Autodesk Inventor part; units mm, degrees
(part 4 of 8)
  arc A302 (101.3786, 36.5166) -> (101.4167, 36.5166) centre (101.3976, 36.5166) ccw
  arc A303 (101.1627, 36.7706) -> (101.1627, 36.7325) centre (101.1627, 36.7516) ccw
  arc A304 (101.1627, 36.7515) -> (100.8756, 36.5427) centre (101.1627, 36.4497) ccw
  arc A305 (101.1627, 36.7325) -> (101.1627, 36.7706) centre (101.1627, 36.7516) ccw
  arc A306 (100.8574, 36.5486) -> (100.8937, 36.5368) centre (100.8756, 36.5427) ccw
  arc A307 (101.3194, 36.3338) -> (101.3977, 36.5166) centre (101.1452, 36.5166) ccw
  arc A308 (101.3062, 36.3476) -> (101.3325, 36.32) centre (101.3194, 36.3338) ccw
  arc A309 (101.4167, 36.5166) -> (101.3786, 36.5166) centre (101.3976, 36.5166) ccw
  line L109 (101.3194, 36.3338) -> (100.8756, 35.8117)
  arc A310 (100.8611, 35.8241) -> (100.8901, 35.7994) centre (100.8756, 35.8118) ccw
  arc A311 (101.3339, 36.3215) -> (101.3049, 36.3462) centre (101.3194, 36.3338) ccw
  line L110 (100.8756, 35.8117) -> (101.3977, 35.8117)
  arc A312 (101.3977, 35.7927) -> (101.3977, 35.8308) centre (101.3977, 35.8118) ccw
  arc A313 (100.8756, 35.8308) -> (100.8756, 35.7927) centre (100.8756, 35.8118) ccw
  arc A314 (98.4358, 24.7896) -> (98.4358, 40.7896) centre (98.4358, 32.7896) ccw
  arc A315 (98.4358, 40.7896) -> (98.4358, 24.7896) centre (98.4358, 32.7896) ccw
  arc A316 (98.4358, 26.2704) -> (98.4358, 39.3088) centre (98.4358, 32.7896) ccw
  arc A317 (98.4358, 39.3088) -> (98.4358, 26.2704) centre (98.4358, 32.7896) ccw
  arc A318 (98.4358, 23.2896) -> (98.4358, 42.2896) centre (98.4358, 32.7896) ccw
  arc A319 (98.4358, 42.2896) -> (98.4358, 23.2896) centre (98.4358, 32.7896) ccw
  arc A320 (75.8576, 81.3321) -> (77.8576, 81.3321) centre (76.8576, 81.3321) ccw
  arc A321 (75.8893, 81.3321) -> (75.8258, 81.3321) centre (75.8576, 81.3321) ccw
  arc A322 (77.8893, 81.3321) -> (77.8258, 81.3321) centre (77.8576, 81.3321) ccw
  line L111 (73.2973, 78.5852) -> (73.5584, 78.794)
  arc A323 (73.5703, 78.7791) -> (73.5465, 78.8089) centre (73.5584, 78.794) ccw
  arc A324 (73.2854, 78.6) -> (73.3092, 78.5703) centre (73.2973, 78.5851) ccw
  line L112 (73.5584, 78.794) -> (73.5584, 77.8542)
  arc A325 (73.5394, 77.8542) -> (73.5774, 77.8542) centre (73.5584, 77.8542) ccw
  arc A326 (73.5774, 78.794) -> (73.5394, 78.794) centre (73.5584, 78.794) ccw
  line L113 (73.2973, 77.8542) -> (73.8195, 77.8542)
  arc A327 (73.8195, 77.8352) -> (73.8195, 77.8732) centre (73.8195, 77.8542) ccw
  arc A328 (73.2973, 77.8732) -> (73.2973, 77.8352) centre (73.2973, 77.8542) ccw
  arc A329 (79.8195, 78.559) -> (79.5845, 78.794) centre (79.5845, 78.559) ccw
  arc A330 (79.8004, 78.559) -> (79.8385, 78.559) centre (79.8194, 78.559) ccw
  arc A331 (79.5845, 78.813) -> (79.5845, 78.775) centre (79.5845, 78.794) ccw
  arc A332 (79.5845, 78.794) -> (79.2973, 78.5852) centre (79.5844, 78.4922) ccw
  arc A333 (79.5845, 78.775) -> (79.5845, 78.813) centre (79.5845, 78.794) ccw
  arc A334 (79.2792, 78.591) -> (79.3155, 78.5793) centre (79.2973, 78.5851) ccw
  arc A335 (79.7411, 78.3763) -> (79.8195, 78.559) centre (79.5671, 78.5591) ccw
  arc A336 (79.728, 78.3901) -> (79.7543, 78.3625) centre (79.7412, 78.3763) ccw
  arc A337 (79.8385, 78.559) -> (79.8004, 78.5591) centre (79.8194, 78.559) ccw
  line L114 (79.7411, 78.3763) -> (79.2973, 77.8542)
  arc A338 (79.2828, 77.8665) -> (79.3119, 77.8419) centre (79.2973, 77.8542) ccw
  arc A339 (79.7557, 78.364) -> (79.7266, 78.3886) centre (79.7412, 78.3763) ccw
  line L115 (79.2973, 77.8542) -> (79.8195, 77.8542)
  arc A340 (79.8195, 77.8352) -> (79.8195, 77.8732) centre (79.8195, 77.8542) ccw
  arc A341 (79.2973, 77.8732) -> (79.2973, 77.8352) centre (79.2973, 77.8542) ccw
  arc A342 (76.8576, 66.8321) -> (76.8576, 82.8321) centre (76.8576, 74.8321) ccw
  arc A343 (76.8576, 82.8321) -> (76.8576, 66.8321) centre (76.8576, 74.8321) ccw
  arc A344 (76.8576, 68.3129) -> (76.8576, 81.3513) centre (76.8576, 74.8321) ccw
  arc A345 (76.8576, 81.3513) -> (76.8576, 68.3129) centre (76.8576, 74.8321) ccw
  arc A346 (76.8576, 65.3321) -> (76.8576, 84.3321) centre (76.8576, 74.8321) ccw
  arc A347 (97.4424, 81.3321) -> (99.4424, 81.3321) centre (98.4424, 81.3321) ccw
  arc A348 (97.4741, 81.3321) -> (97.4106, 81.3321) centre (97.4424, 81.3321) ccw
  arc A349 (99.4741, 81.3321) -> (99.4106, 81.3321) centre (99.4424, 81.3321) ccw
  line L116 (94.8822, 78.5852) -> (95.1432, 78.794)
  arc A350 (95.1551, 78.7791) -> (95.1313, 78.8089) centre (95.1432, 78.794) ccw
  arc A351 (94.8703, 78.6) -> (94.8941, 78.5703) centre (94.8822, 78.5851) ccw
  line L117 (95.1432, 78.794) -> (95.1432, 77.8542)
  arc A352 (95.1242, 77.8542) -> (95.1623, 77.8542) centre (95.1432, 77.8542) ccw
  arc A353 (95.1623, 78.794) -> (95.1242, 78.794) centre (95.1432, 78.794) ccw
  line L118 (94.8822, 77.8542) -> (95.4043, 77.8542)
  arc A354 (95.4043, 77.8352) -> (95.4043, 77.8732) centre (95.4043, 77.8542) ccw
  arc A355 (94.8822, 77.8732) -> (94.8822, 77.8352) centre (94.8822, 77.8542) ccw
  arc A356 (101.4043, 78.559) -> (101.1693, 78.794) centre (101.1693, 78.559) ccw
  arc A357 (101.3852, 78.559) -> (101.4233, 78.559) centre (101.4043, 78.559) ccw
  arc A358 (101.1693, 78.813) -> (101.1693, 78.775) centre (101.1693, 78.794) ccw
  arc A359 (101.1693, 78.794) -> (100.8822, 78.5852) centre (101.1693, 78.4922) ccw
  arc A360 (101.1693, 78.775) -> (101.1693, 78.813) centre (101.1693, 78.794) ccw
  arc A361 (100.864, 78.591) -> (100.9003, 78.5793) centre (100.8821, 78.5851) ccw
  arc A362 (101.326, 78.3763) -> (101.4043, 78.559) centre (101.1519, 78.559) ccw
  arc A363 (101.3128, 78.3901) -> (101.3391, 78.3625) centre (101.326, 78.3763) ccw
  arc A364 (101.4233, 78.559) -> (101.3852, 78.5591) centre (101.4043, 78.559) ccw
  line L119 (101.326, 78.3763) -> (100.8822, 77.8542)
  arc A365 (100.8677, 77.8665) -> (100.8967, 77.8419) centre (100.8822, 77.8542) ccw
  arc A366 (101.3405, 78.364) -> (101.3114, 78.3886) centre (101.326, 78.3763) ccw
  line L120 (100.8822, 77.8542) -> (101.4043, 77.8542)
  arc A367 (101.4043, 77.8352) -> (101.4043, 77.8732) centre (101.4043, 77.8542) ccw
  arc A368 (100.8822, 77.8732) -> (100.8822, 77.8352) centre (100.8822, 77.8542) ccw
  arc A369 (98.4424, 66.8321) -> (98.4424, 82.8321) centre (98.4424, 74.8321) ccw
  arc A370 (98.4424, 82.8321) -> (98.4424, 66.8321) centre (98.4424, 74.8321) ccw
  arc A371 (98.4424, 68.3129) -> (98.4424, 81.3513) centre (98.4424, 74.8321) ccw
  arc A372 (98.4424, 81.3513) -> (98.4424, 68.3129) centre (98.4424, 74.8321) ccw
  arc A373 (98.4424, 65.3321) -> (98.4424, 84.3321) centre (98.4424, 74.8321) ccw
  arc A374 (98.4424, 84.3321) -> (98.4424, 65.3321) centre (98.4424, 74.8321) ccw
  arc A375 (34.6796, 5.5886) -> (32.6796, 5.5886) centre (33.6796, 5.5886) ccw
  arc A376 (34.6479, 5.5886) -> (34.7114, 5.5886) centre (34.6796, 5.5886) ccw
  arc A377 (32.6479, 5.5886) -> (32.7114, 5.5886) centre (32.6796, 5.5886) ccw
  line L121 (38.7177, 11.8577) -> (38.9788, 12.0665)
  arc A378 (38.9907, 12.0517) -> (38.9669, 12.0814) centre (38.9788, 12.0665) ccw
  arc A379 (38.7058, 11.8726) -> (38.7296, 11.8428) centre (38.7177, 11.8577) ccw
  line L122 (38.9788, 12.0665) -> (38.9788, 11.1267)
  arc A380 (38.9597, 11.1267) -> (38.9978, 11.1267) centre (38.9787, 11.1267) ccw
  arc A381 (38.9978, 12.0665) -> (38.9597, 12.0665) centre (38.9787, 12.0665) ccw
  line L123 (38.7177, 11.1267) -> (39.2398, 11.1267)
  arc A382 (39.2398, 11.1077) -> (39.2398, 11.1458) centre (39.2398, 11.1268) ccw
  arc A383 (38.7177, 11.1458) -> (38.7177, 11.1077) centre (38.7177, 11.1268) ccw
  arc A384 (36.2398, 16.8316) -> (36.0049, 17.0665) centre (36.0049, 16.8316) ccw
  arc A385 (36.2208, 16.8316) -> (36.2589, 16.8316) centre (36.2398, 16.8316) ccw
  arc A386 (36.0049, 17.0856) -> (36.0049, 17.0475) centre (36.0049, 17.0665) ccw
  arc A387 (36.0049, 17.0665) -> (35.7177, 16.8577) centre (36.0048, 16.7647) ccw
  arc A388 (36.0049, 17.0475) -> (36.0049, 17.0856) centre (36.0049, 17.0665) ccw
  arc A389 (35.6996, 16.8636) -> (35.7358, 16.8518) centre (35.7177, 16.8577) ccw
  arc A390 (36.1615, 16.6488) -> (36.2398, 16.8316) centre (35.9873, 16.8316) ccw
  arc A391 (36.1484, 16.6626) -> (36.1746, 16.635) centre (36.1615, 16.6488) ccw
  arc A392 (36.2589, 16.8316) -> (36.2208, 16.8316) centre (36.2398, 16.8316) ccw
  line L124 (36.1615, 16.6488) -> (35.7177, 16.1267)
  arc A393 (35.7032, 16.1391) -> (35.7322, 16.1144) centre (35.7177, 16.1268) ccw
  arc A394 (36.176, 16.6365) -> (36.147, 16.6612) centre (36.1615, 16.6489) ccw
  line L125 (35.7177, 16.1267) -> (36.2398, 16.1267)
  arc A395 (36.2398, 16.1077) -> (36.2398, 16.1458) centre (36.2398, 16.1268) ccw
  arc A396 (35.7177, 16.1458) -> (35.7177, 16.1077) centre (35.7177, 16.1268) ccw
  line L126 (32.7177, 11.1267) -> (32.9788, 11.1267)
  arc A397 (32.9788, 11.1077) -> (32.9788, 11.1458) centre (32.9788, 11.1268) ccw
  arc A398 (32.7177, 11.1458) -> (32.7177, 11.1077) centre (32.7177, 11.1268) ccw
  arc A399 (32.9788, 11.1267) -> (32.9788, 11.6488) centre (32.9788, 11.3878) ccw
  arc A400 (32.9788, 11.1458) -> (32.9788, 11.1077) centre (32.9788, 11.1268) ccw
  arc A401 (32.9788, 11.6679) -> (32.9788, 11.6298) centre (32.9788, 11.6488) ccw
  line L127 (32.7177, 12.0665) -> (33.031, 12.0665)
  arc A402 (33.031, 12.0475) -> (33.031, 12.0856) centre (33.031, 12.0665) ccw
  arc A403 (32.7177, 12.0856) -> (32.7177, 12.0475) centre (32.7177, 12.0665) ccw
  arc A404 (33.031, 11.6488) -> (33.031, 12.0665) centre (33.031, 11.8576) ccw
  arc A405 (33.031, 11.6679) -> (33.031, 11.6298) centre (33.031, 11.6488) ccw
  arc A406 (33.031, 12.0856) -> (33.031, 12.0475) centre (33.031, 12.0665) ccw
  line L128 (33.031, 11.6488) -> (32.8221, 11.6488)
  arc A407 (32.8221, 11.6679) -> (32.8221, 11.6298) centre (32.8221, 11.6488) ccw
  arc A408 (33.031, 11.6298) -> (33.031, 11.6679) centre (33.031, 11.6488) ccw
  arc A409 (33.6796, 4.0886) -> (33.6796, 20.0886) centre (33.6796, 12.0886) ccw
  arc A410 (33.6796, 20.0886) -> (33.6796, 4.0886) centre (33.6796, 12.0886) ccw
  arc A411 (33.6796, 5.5694) -> (33.6796, 18.6078) centre (33.6796, 12.0886) ccw
  arc A412 (33.6796, 18.6078) -> (33.6796, 5.5694) centre (33.6796, 12.0886) ccw
  arc A413 (33.6796, 2.5886) -> (33.6796, 21.5886) centre (33.6796, 12.0886) ccw
  arc A414 (33.6796, 21.5886) -> (33.6796, 2.5886) centre (33.6796, 12.0886) ccw
  arc A415 (32.6842, 60.4569) -> (34.6842, 60.4569) centre (33.6842, 60.4569) ccw
  arc A416 (32.716, 60.4569) -> (32.6525, 60.4569) centre (32.6843, 60.4569) ccw
  arc A417 (34.716, 60.4569) -> (34.6525, 60.4569) centre (34.6843, 60.4569) ccw
  line L129 (28.624, 55.21) -> (28.8851, 55.4188)
  arc A418 (28.897, 55.4039) -> (28.8732, 55.4337) centre (28.8851, 55.4188) ccw
  arc A419 (28.6121, 55.2248) -> (28.6359, 55.1951) centre (28.624, 55.2099) ccw
  line L130 (28.8851, 55.4188) -> (28.8851, 54.479)
  arc A420 (28.866, 54.479) -> (28.9041, 54.479) centre (28.8851, 54.479) ccw
  arc A421 (28.9041, 55.4188) -> (28.866, 55.4188) centre (28.8851, 55.4188) ccw
  line L131 (28.624, 54.479) -> (29.1461, 54.479)
  arc A422 (29.1461, 54.46) -> (29.1461, 54.4981) centre (29.1461, 54.4791) ccw
  arc A423 (28.624, 54.4981) -> (28.624, 54.46) centre (28.624, 54.4791) ccw
  arc A424 (29.1461, 53.1839) -> (28.9112, 53.4188) centre (28.9112, 53.1839) ccw
  arc A425 (29.1271, 53.1839) -> (29.1652, 53.1839) centre (29.1461, 53.1839) ccw
  arc A426 (28.9112, 53.4379) -> (28.9112, 53.3998) centre (28.9112, 53.4189) ccw
  arc A427 (28.9112, 53.4188) -> (28.624, 53.21) centre (28.9111, 53.117) ccw
  arc A428 (28.9112, 53.3998) -> (28.9112, 53.4379) centre (28.9112, 53.4189) ccw
  arc A429 (28.6059, 53.2158) -> (28.6421, 53.2041) centre (28.624, 53.2099) ccw
  arc A430 (29.0678, 53.0011) -> (29.1461, 53.1839) centre (28.8936, 53.1839) ccw
  arc A431 (29.0547, 53.0149) -> (29.0809, 52.9873) centre (29.0678, 53.0011) ccw
  arc A432 (29.1652, 53.1839) -> (29.1271, 53.1839) centre (29.1461, 53.1839) ccw
  line L132 (29.0678, 53.0011) -> (28.624, 52.479)
  arc A433 (28.6095, 52.4914) -> (28.6385, 52.4667) centre (28.624, 52.4791) ccw
  arc A434 (29.0823, 52.9888) -> (29.0533, 53.0135) centre (29.0678, 53.0011) ccw
  line L133 (28.624, 52.479) -> (29.1461, 52.479)
  arc A435 (29.1461, 52.46) -> (29.1461, 52.4981) centre (29.1461, 52.4791) ccw
  arc A436 (28.624, 52.4981) -> (28.624, 52.46) centre (28.624, 52.4791) ccw
  line L134 (38.124, 52.479) -> (38.3851, 52.479)
  arc A437 (38.3851, 52.46) -> (38.3851, 52.4981) centre (38.3851, 52.4791) ccw
  arc A438 (38.124, 52.4981) -> (38.124, 52.46) centre (38.124, 52.4791) ccw
  arc A439 (38.3851, 52.479) -> (38.3851, 53.0011) centre (38.3851, 52.74) ccw
  arc A440 (38.3851, 52.4981) -> (38.3851, 52.46) centre (38.3851, 52.4791) ccw
  arc A441 (38.3851, 53.0202) -> (38.3851, 52.9821) centre (38.3851, 53.0012) ccw
  line L135 (38.124, 53.4188) -> (38.4373, 53.4188)
  arc A442 (38.4373, 53.3998) -> (38.4373, 53.4379) centre (38.4373, 53.4189) ccw
  arc A443 (38.124, 53.4379) -> (38.124, 53.3998) centre (38.124, 53.4189) ccw
  arc A444 (38.4373, 53.0011) -> (38.4373, 53.4188) centre (38.4373, 53.2099) ccw
  arc A445 (38.4373, 53.0202) -> (38.4373, 52.9821) centre (38.4373, 53.0012) ccw
  arc A446 (38.4373, 53.4379) -> (38.4373, 53.3998) centre (38.4373, 53.4189) ccw
  line L136 (38.4373, 53.0011) -> (38.2284, 53.0011)
  arc A447 (38.2284, 53.0202) -> (38.2284, 52.9821) centre (38.2284, 53.0012) ccw
  arc A448 (38.4373, 52.9821) -> (38.4373, 53.0202) centre (38.4373, 53.0012) ccw
  line L137 (38.3328, 55.4188) -> (38.124, 54.6879)
  arc A449 (38.1057, 54.6931) -> (38.1423, 54.6826) centre (38.124, 54.6879) ccw
  arc A450 (38.3512, 55.4136) -> (38.3145, 55.424) centre (38.3329, 55.4188) ccw
  line L138 (38.124, 54.6879) -> (38.6461, 54.6879)
  arc A451 (38.6461, 54.6688) -> (38.6461, 54.7069) centre (38.6461, 54.6879) ccw
  arc A452 (38.124, 54.7069) -> (38.124, 54.6688) centre (38.124, 54.6879) ccw
  line L139 (38.4895, 54.8967) -> (38.4895, 54.479)
  arc A453 (38.4704, 54.479) -> (38.5085, 54.479) centre (38.4894, 54.479) ccw
  arc A454 (38.5085, 54.8967) -> (38.4704, 54.8967) centre (38.4894, 54.8967) ccw
  arc A455 (33.6842, 45.9569) -> (33.6842, 61.9569) centre (33.6842, 53.9569) ccw
  arc A456 (33.6842, 61.9569) -> (33.6842, 45.9569) centre (33.6842, 53.9569) ccw
  arc A457 (33.6842, 47.4377) -> (33.6842, 60.4761) centre (33.6842, 53.9569) ccw
  arc A458 (33.6842, 60.4761) -> (33.6842, 47.4377) centre (33.6842, 53.9569) ccw
  arc A459 (33.6842, 44.4569) -> (33.6842, 63.4569) centre (33.6842, 53.9569) ccw
  arc A460 (33.6842, 63.4569) -> (33.6842, 44.4569) centre (33.6842, 53.9569) ccw
  arc A461 (11.0477, 60.2972) -> (13.0477, 60.2972) centre (12.0477, 60.2972) ccw
  arc A462 (11.0794, 60.2972) -> (11.0159, 60.2972) centre (11.0477, 60.2972) ccw
  arc A463 (13.0794, 60.2972) -> (13.0159, 60.2972) centre (13.0477, 60.2972) ccw
  line L140 (6.4875, 54.5503) -> (6.7485, 54.7591)
  arc A464 (6.7604, 54.7442) -> (6.7366, 54.774) centre (6.7485, 54.7591) ccw
  arc A465 (6.4756, 54.5651) -> (6.4994, 54.5354) centre (6.4875, 54.5503) ccw
  line L141 (6.7485, 54.7591) -> (6.7485, 53.8193)
  arc A466 (6.7295, 53.8193) -> (6.7676, 53.8193) centre (6.7485, 53.8193) ccw
  arc A467 (6.7676, 54.7591) -> (6.7295, 54.7591) centre (6.7485, 54.7591) ccw
  line L142 (6.4875, 53.8193) -> (7.0096, 53.8193)
  arc A468 (7.0096, 53.8003) -> (7.0096, 53.8384) centre (7.0096, 53.8194) ccw
  arc A469 (6.4875, 53.8384) -> (6.4875, 53.8003) centre (6.4875, 53.8194) ccw
  arc A470 (10.0096, 49.5242) -> (9.7746, 49.7591) centre (9.7746, 49.5241) ccw
  arc A471 (9.9905, 49.5242) -> (10.0286, 49.5242) centre (10.0096, 49.5242) ccw
  arc A472 (9.7746, 49.7782) -> (9.7746, 49.7401) centre (9.7746, 49.7592) ccw
  arc A473 (9.7746, 49.7591) -> (9.4875, 49.5503) centre (9.7746, 49.4573) ccw
  arc A474 (9.7746, 49.7401) -> (9.7746, 49.7781) centre (9.7746, 49.7591) ccw
  arc A475 (9.4694, 49.5561) -> (9.5056, 49.5444) centre (9.4875, 49.5503) ccw
  arc A476 (9.9313, 49.3414) -> (10.0096, 49.5242) centre (9.7571, 49.5242) ccw
  arc A477 (9.9181, 49.3552) -> (9.9444, 49.3276) centre (9.9313, 49.3414) ccw
  arc A478 (10.0286, 49.5241) -> (9.9905, 49.5242) centre (10.0096, 49.5242) ccw
  line L143 (9.9313, 49.3414) -> (9.4875, 48.8193)
  arc A479 (9.473, 48.8316) -> (9.502, 48.807) centre (9.4875, 48.8193) ccw
  arc A480 (9.9458, 49.3291) -> (9.9168, 49.3537) centre (9.9313, 49.3414) ccw
  line L144 (9.4875, 48.8193) -> (10.0096, 48.8193)
  arc A481 (10.0096, 48.8003) -> (10.0096, 48.8384) centre (10.0096, 48.8194) ccw
  arc A482 (9.4875, 48.8384) -> (9.4875, 48.8003) centre (9.4875, 48.8194) ccw
  line L145 (12.4875, 53.8193) -> (12.7485, 53.8193)
  arc A483 (12.7485, 53.8003) -> (12.7485, 53.8384) centre (12.7485, 53.8194) ccw
  arc A484 (12.4875, 53.8384) -> (12.4875, 53.8003) centre (12.4875, 53.8194) ccw
  arc A485 (12.7485, 53.8193) -> (12.7485, 54.3414) centre (12.7485, 54.0803) ccw
  arc A486 (12.7485, 53.8384) -> (12.7485, 53.8003) centre (12.7485, 53.8194) ccw
  arc A487 (12.7485, 54.3605) -> (12.7485, 54.3224) centre (12.7485, 54.3415) ccw
  line L146 (12.4875, 54.7591) -> (12.8007, 54.7591)
  arc A488 (12.8007, 54.7401) -> (12.8007, 54.7782) centre (12.8007, 54.7592) ccw
  arc A489 (12.4875, 54.7782) -> (12.4875, 54.7401) centre (12.4875, 54.7592) ccw
  arc A490 (12.8007, 54.3414) -> (12.8007, 54.7591) centre (12.8007, 54.5502) ccw
  arc A491 (12.8007, 54.3605) -> (12.8007, 54.3224) centre (12.8007, 54.3415) ccw
  arc A492 (12.8007, 54.7782) -> (12.8007, 54.7401) centre (12.8007, 54.7592) ccw
  line L147 (12.8007, 54.3414) -> (12.5919, 54.3414)
  arc A493 (12.5919, 54.3605) -> (12.5919, 54.3224) centre (12.5919, 54.3415) ccw
  arc A494 (12.8007, 54.3224) -> (12.8007, 54.3605) centre (12.8007, 54.3415) ccw
  arc A495 (12.0477, 45.7972) -> (12.0477, 61.7972) centre (12.0477, 53.7972) ccw
  arc A496 (12.0477, 61.7972) -> (12.0477, 45.7972) centre (12.0477, 53.7972) ccw
  arc A497 (12.0477, 47.278) -> (12.0477, 60.3164) centre (12.0477, 53.7972) ccw
  arc A498 (12.0477, 60.3164) -> (12.0477, 47.278) centre (12.0477, 53.7972) ccw
  arc A499 (12.0477, 44.2972) -> (12.0477, 63.2972) centre (12.0477, 53.7972) ccw
  arc A500 (12.0477, 63.2972) -> (12.0477, 44.2972) centre (12.0477, 53.7972) ccw
  arc A501 (13.085, 5.5469) -> (11.085, 5.5469) centre (12.085, 5.5469) ccw
  arc A502 (13.0532, 5.5469) -> (13.1167, 5.5469) centre (13.0849, 5.5469) ccw
  arc A503 (11.0532, 5.5469) -> (11.1167, 5.5469) centre (11.0849, 5.5469) ccw
  line L148 (17.1231, 11.816) -> (17.3842, 12.0248)
  arc A504 (17.3961, 12.0099) -> (17.3722, 12.0397) centre (17.3841, 12.0248) ccw
  arc A505 (17.1112, 11.8308) -> (17.135, 11.8011) centre (17.1231, 11.816) ccw
  line L149 (17.3842, 12.0248) -> (17.3842, 11.085)
  arc A506 (17.3651, 11.085) -> (17.4032, 11.085) centre (17.3841, 11.085) ccw
  arc A507 (17.4032, 12.0248) -> (17.3651, 12.0248) centre (17.3841, 12.0248) ccw
  line L150 (17.1231, 11.085) -> (17.6452, 11.085)
  arc A508 (17.6452, 11.066) -> (17.6452, 11.1041) centre (17.6452, 11.0851) ccw
  arc A509 (17.1231, 11.1041) -> (17.1231, 11.066) centre (17.1231, 11.0851) ccw
  arc A510 (14.6452, 16.7899) -> (14.4103, 17.0248) centre (14.4103, 16.7899) ccw
  arc A511 (14.6262, 16.7899) -> (14.6643, 16.7899) centre (14.6453, 16.7899) ccw
  arc A512 (14.4103, 17.0439) -> (14.4103, 17.0058) centre (14.4103, 17.0249) ccw
  arc A513 (14.4103, 17.0248) -> (14.1231, 16.816) centre (14.4102, 16.723) ccw
  arc A514 (14.4103, 17.0058) -> (14.4103, 17.0439) centre (14.4103, 17.0249) ccw
  arc A515 (14.105, 16.8218) -> (14.1412, 16.8101) centre (14.1231, 16.816) ccw
  arc A516 (14.5669, 16.6071) -> (14.6452, 16.7899) centre (14.3927, 16.7899) ccw
  arc A517 (14.5538, 16.6209) -> (14.58, 16.5933) centre (14.5669, 16.6071) ccw
  arc A518 (14.6643, 16.7899) -> (14.6262, 16.7899) centre (14.6453, 16.7899) ccw
  line L151 (14.5669, 16.6071) -> (14.1231, 16.085)
  arc A519 (14.1086, 16.0974) -> (14.1376, 16.0727) centre (14.1231, 16.0851) ccw
  arc A520 (14.5814, 16.5948) -> (14.5524, 16.6195) centre (14.5669, 16.6071) ccw
  line L152 (14.1231, 16.085) -> (14.6452, 16.085)
  arc A521 (14.6452, 16.066) -> (14.6452, 16.1041) centre (14.6452, 16.0851) ccw
  arc A522 (14.1231, 16.1041) -> (14.1231, 16.066) centre (14.1231, 16.0851) ccw
  line L153 (11.1231, 11.085) -> (11.3841, 11.085)
  arc A523 (11.3841, 11.066) -> (11.3841, 11.1041) centre (11.3841, 11.0851) ccw
  arc A524 (11.1231, 11.1041) -> (11.1231, 11.066) centre (11.1231, 11.0851) ccw
  arc A525 (11.3841, 11.085) -> (11.3841, 11.6071) centre (11.3841, 11.3461) ccw
  arc A526 (11.3841, 11.1041) -> (11.3841, 11.066) centre (11.3841, 11.0851) ccw
  arc A527 (11.3841, 11.6262) -> (11.3841, 11.5881) centre (11.3841, 11.6072) ccw
  line L154 (11.1231, 12.0248) -> (11.4364, 12.0248)
  arc A528 (11.4364, 12.0058) -> (11.4364, 12.0439) centre (11.4364, 12.0249) ccw
  arc A529 (11.1231, 12.0439) -> (11.1231, 12.0058) centre (11.1231, 12.0249) ccw
  arc A530 (11.4364, 11.6071) -> (11.4364, 12.0248) centre (11.4364, 11.816) ccw
  arc A531 (11.4364, 11.6262) -> (11.4364, 11.5881) centre (11.4364, 11.6072) ccw
  arc A532 (11.4364, 12.0439) -> (11.4364, 12.0058) centre (11.4364, 12.0249) ccw
  line L155 (11.4364, 11.6071) -> (11.2275, 11.6071)
  arc A533 (11.2275, 11.6262) -> (11.2275, 11.5881) centre (11.2275, 11.6072) ccw
  arc A534 (11.4364, 11.5881) -> (11.4364, 11.6262) centre (11.4364, 11.6072) ccw
  arc A535 (12.085, 4.0469) -> (12.085, 20.0469) centre (12.085, 12.0469) ccw
  arc A536 (12.085, 20.0469) -> (12.085, 4.0469) centre (12.085, 12.0469) ccw
  arc A537 (12.085, 5.5277) -> (12.085, 18.5661) centre (12.085, 12.0469) ccw
  arc A538 (12.085, 18.5661) -> (12.085, 5.5277) centre (12.085, 12.0469) ccw
  arc A539 (12.085, 2.5469) -> (12.085, 21.5469) centre (12.085, 12.0469) ccw
  arc A540 (12.085, 21.5469) -> (12.085, 2.5469) centre (12.085, 12.0469) ccw
  arc A541 (56.3493, 5.6412) -> (54.3493, 5.6412) centre (55.3493, 5.6412) ccw
  arc A542 (56.3175, 5.6412) -> (56.381, 5.6412) centre (56.3492, 5.6412) ccw
  arc A543 (54.3175, 5.6412) -> (54.381, 5.6412) centre (54.3492, 5.6412) ccw
  line L156 (59.8874, 11.4103) -> (60.1485, 11.6191)
  arc A544 (60.1604, 11.6042) -> (60.1365, 11.634) centre (60.1485, 11.6191) ccw
  arc A545 (59.8755, 11.4251) -> (59.8993, 11.3954) centre (59.8874, 11.4103) ccw
  line L157 (60.1485, 11.6191) -> (60.1485, 10.6793)
  arc A546 (60.1294, 10.6793) -> (60.1675, 10.6793) centre (60.1485, 10.6793) ccw
  arc A547 (60.1675, 11.6191) -> (60.1294, 11.6191) centre (60.1485, 11.6191) ccw
  line L158 (59.8874, 10.6793) -> (60.4095, 10.6793)
  arc A548 (60.4095, 10.6603) -> (60.4095, 10.6984) centre (60.4095, 10.6794) ccw
  arc A549 (59.8874, 10.6984) -> (59.8874, 10.6603) centre (59.8874, 10.6794) ccw
  arc A550 (60.4095, 13.3841) -> (60.1746, 13.6191) centre (60.1745, 13.3841) ccw
  arc A551 (60.3905, 13.3841) -> (60.4286, 13.3841) centre (60.4096, 13.3841) ccw
  arc A552 (60.1746, 13.6382) -> (60.1746, 13.6001) centre (60.1746, 13.6191) ccw
  arc A553 (60.1746, 13.6191) -> (59.8874, 13.4103) centre (60.1745, 13.3173) ccw
  arc A554 (60.1746, 13.6001) -> (60.1746, 13.6381) centre (60.1746, 13.6191) ccw
  arc A555 (59.8693, 13.4161) -> (59.9055, 13.4044) centre (59.8874, 13.4103) ccw
  arc A556 (60.3312, 13.2014) -> (60.4095, 13.3841) centre (60.1571, 13.3841) ccw
  arc A557 (60.3181, 13.2152) -> (60.3443, 13.1876) centre (60.3312, 13.2014) ccw
  arc A558 (60.4286, 13.3841) -> (60.3905, 13.3842) centre (60.4096, 13.3842) ccw
  line L159 (60.3312, 13.2014) -> (59.8874, 12.6793)
  arc A559 (59.8729, 12.6916) -> (59.9019, 12.667) centre (59.8874, 12.6793) ccw
  arc A560 (60.3457, 13.1891) -> (60.3167, 13.2137) centre (60.3312, 13.2014) ccw
  line L160 (59.8874, 12.6793) -> (60.4095, 12.6793)
  arc A561 (60.4095, 12.6603) -> (60.4095, 12.6984) centre (60.4095, 12.6793) ccw
  arc A562 (59.8874, 12.6984) -> (59.8874, 12.6603) centre (59.8874, 12.6793) ccw
  line L161 (50.3874, 12.6793) -> (50.6485, 12.6793)
  arc A563 (50.6485, 12.6603) -> (50.6485, 12.6984) centre (50.6485, 12.6793) ccw
  arc A564 (50.3874, 12.6984) -> (50.3874, 12.6603) centre (50.3874, 12.6793) ccw
  arc A565 (50.6485, 12.6793) -> (50.6485, 13.2014) centre (50.6485, 12.9404) ccw
  arc A566 (50.6485, 12.6984) -> (50.6485, 12.6603) centre (50.6485, 12.6793) ccw
  arc A567 (50.6485, 13.2205) -> (50.6485, 13.1824) centre (50.6485, 13.2015) ccw
  line L162 (50.3874, 13.6191) -> (50.7007, 13.6191)
  arc A568 (50.7007, 13.6001) -> (50.7007, 13.6382) centre (50.7007, 13.6191) ccw
  arc A569 (50.3874, 13.6382) -> (50.3874, 13.6001) centre (50.3874, 13.6191) ccw
  arc A570 (50.7007, 13.2014) -> (50.7007, 13.6191) centre (50.7007, 13.4103) ccw
  arc A571 (50.7007, 13.2205) -> (50.7007, 13.1824) centre (50.7007, 13.2015) ccw
  arc A572 (50.7007, 13.6382) -> (50.7007, 13.6001) centre (50.7007, 13.6191) ccw
  line L163 (50.7007, 13.2014) -> (50.4918, 13.2014)
  arc A573 (50.4918, 13.2205) -> (50.4918, 13.1824) centre (50.4918, 13.2015) ccw
  arc A574 (50.7007, 13.1824) -> (50.7007, 13.2205) centre (50.7007, 13.2015) ccw
  line L164 (50.5962, 11.6191) -> (50.3874, 10.8881)
  arc A575 (50.3691, 10.8934) -> (50.4057, 10.8829) centre (50.3874, 10.8882) ccw
  arc A576 (50.6146, 11.6139) -> (50.5779, 11.6243) centre (50.5963, 11.6191) ccw
  line L165 (50.3874, 10.8881) -> (50.9095, 10.8881)
  arc A577 (50.9095, 10.8691) -> (50.9095, 10.9072) centre (50.9095, 10.8882) ccw
  arc A578 (50.3874, 10.9072) -> (50.3874, 10.8691) centre (50.3874, 10.8882) ccw
  line L166 (50.7529, 11.097) -> (50.7529, 10.6793)
  arc A579 (50.7338, 10.6793) -> (50.7719, 10.6793) centre (50.7529, 10.6793) ccw
  arc A580 (50.7719, 11.097) -> (50.7338, 11.097) centre (50.7529, 11.097) ccw
  arc A581 (55.3493, 4.1412) -> (55.3493, 20.1412) centre (55.3493, 12.1412) ccw
  arc A582 (55.3493, 20.1412) -> (55.3493, 4.1412) centre (55.3493, 12.1412) ccw
  arc A583 (55.3493, 5.622) -> (55.3493, 18.6604) centre (55.3493, 12.1412) ccw
  arc A584 (55.3493, 18.6604) -> (55.3493, 5.622) centre (55.3493, 12.1412) ccw
  arc A585 (55.3493, 2.6412) -> (55.3493, 21.6412) centre (55.3493, 12.1412) ccw
  arc A586 (55.3493, 21.6412) -> (55.3493, 2.6412) centre (55.3493, 12.1412) ccw
  arc A587 (32.5609, 81.4119) -> (34.5609, 81.4119) centre (33.5609, 81.4119) ccw
  arc A588 (32.5927, 81.4119) -> (32.5292, 81.4119) centre (32.561, 81.4119) ccw
  arc A589 (34.5927, 81.4119) -> (34.5292, 81.4119) centre (34.561, 81.4119) ccw
  line L167 (28.5007, 76.165) -> (28.7618, 76.3738)
  arc A590 (28.7737, 76.3589) -> (28.7499, 76.3887) centre (28.7618, 76.3738) ccw
  arc A591 (28.4888, 76.1798) -> (28.5126, 76.1501) centre (28.5007, 76.165) ccw
  line L168 (28.7618, 76.3738) -> (28.7618, 75.434)
  arc A592 (28.7427, 75.434) -> (28.7808, 75.434) centre (28.7617, 75.434) ccw
  arc A593 (28.7808, 76.3738) -> (28.7427, 76.3738) centre (28.7617, 76.3738) ccw
  line L169 (28.5007, 75.434) -> (29.0228, 75.434)
  arc A594 (29.0228, 75.415) -> (29.0228, 75.4531) centre (29.0228, 75.4341) ccw
  arc A595 (28.5007, 75.4531) -> (28.5007, 75.415) centre (28.5007, 75.4341) ccw
  arc A596 (29.0228, 74.1389) -> (28.7879, 74.3738) centre (28.7879, 74.1389) ccw
  arc A597 (29.0038, 74.1389) -> (29.0419, 74.1389) centre (29.0228, 74.1389) ccw
  arc A598 (28.7879, 74.3929) -> (28.7879, 74.3548) centre (28.7879, 74.3739) ccw
  arc A599 (28.7879, 74.3738) -> (28.5007, 74.165) centre (28.7878, 74.072) ccw
  arc A600 (28.7879, 74.3548) -> (28.7879, 74.3929) centre (28.7879, 74.3739) ccw
  arc A601 (28.4826, 74.1708) -> (28.5188, 74.1591) centre (28.5007, 74.165) ccw
  arc A602 (28.9445, 73.9561) -> (29.0228, 74.1389) centre (28.7703, 74.1389) ccw
  arc A603 (28.9314, 73.9699) -> (28.9576, 73.9423) centre (28.9445, 73.9561) ccw
  arc A604 (29.0419, 74.1389) -> (29.0038, 74.1389) centre (29.0228, 74.1389) ccw
  line L170 (28.9445, 73.9561) -> (28.5007, 73.434)
  arc A605 (28.4862, 73.4464) -> (28.5152, 73.4217) centre (28.5007, 73.4341) ccw
  arc A606 (28.959, 73.9438) -> (28.93, 73.9685) centre (28.9445, 73.9562) ccw
  line L171 (28.5007, 73.434) -> (29.0228, 73.434)
  arc A607 (29.0228, 73.415) -> (29.0228, 73.4531) centre (29.0228, 73.4341) ccw
  arc A608 (28.5007, 73.4531) -> (28.5007, 73.415) centre (28.5007, 73.4341) ccw
  line L172 (38.0007, 73.434) -> (38.2618, 73.434)
  arc A609 (38.2618, 73.415) -> (38.2618, 73.4531) centre (38.2618, 73.4341) ccw
  arc A610 (38.0007, 73.4531) -> (38.0007, 73.415) centre (38.0007, 73.4341) ccw
  arc A611 (38.2618, 73.434) -> (38.2618, 73.9561) centre (38.2618, 73.6951) ccw
  arc A612 (38.2618, 73.4531) -> (38.2618, 73.415) centre (38.2618, 73.4341) ccw
  arc A613 (38.2618, 73.9752) -> (38.2618, 73.9371) centre (38.2618, 73.9562) ccw
  line L173 (38.0007, 74.3738) -> (38.314, 74.3738)
  arc A614 (38.314, 74.3548) -> (38.314, 74.3929) centre (38.314, 74.3739) ccw
  arc A615 (38.0007, 74.3929) -> (38.0007, 74.3548) centre (38.0007, 74.3739) ccw
  arc A616 (38.314, 73.9561) -> (38.314, 74.3738) centre (38.314, 74.165) ccw
  arc A617 (38.314, 73.9752) -> (38.314, 73.9371) centre (38.314, 73.9562) ccw
  arc A618 (38.314, 74.3929) -> (38.314, 74.3548) centre (38.314, 74.3739) ccw
  line L174 (38.314, 73.9561) -> (38.1051, 73.9561)
  arc A619 (38.1051, 73.9752) -> (38.1051, 73.9371) centre (38.1051, 73.9562) ccw
  arc A620 (38.314, 73.9371) -> (38.314, 73.9752) centre (38.314, 73.9562) ccw
  line L175 (38.2096, 76.3738) -> (38.0007, 75.6429)
  arc A621 (37.9824, 75.6481) -> (38.019, 75.6376) centre (38.0007, 75.6429) ccw
  arc A622 (38.2279, 76.3686) -> (38.1912, 76.379) centre (38.2096, 76.3738) ccw
  line L176 (38.0007, 75.6429) -> (38.5228, 75.6429)
  arc A623 (38.5228, 75.6238) -> (38.5228, 75.6619) centre (38.5228, 75.6429) ccw
  arc A624 (38.0007, 75.6619) -> (38.0007, 75.6238) centre (38.0007, 75.6429) ccw
  line L177 (38.3662, 75.8517) -> (38.3662, 75.434)
  arc A625 (38.3471, 75.434) -> (38.3852, 75.434) centre (38.3662, 75.434) ccw
  arc A626 (38.3852, 75.8517) -> (38.3471, 75.8517) centre (38.3662, 75.8517) ccw
  arc A627 (33.5609, 66.9119) -> (33.5609, 82.9119) centre (33.5609, 74.9119) ccw
  arc A628 (33.5609, 82.9119) -> (33.5609, 66.9119) centre (33.5609, 74.9119) ccw
  arc A629 (33.5609, 68.3927) -> (33.5609, 81.4311) centre (33.5609, 74.9119) ccw
  arc A630 (33.5609, 81.4311) -> (33.5609, 68.3927) centre (33.5609, 74.9119) ccw
  arc A631 (33.5609, 65.4119) -> (33.5609, 84.4119) centre (33.5609, 74.9119) ccw
  arc A632 (33.5609, 84.4119) -> (33.5609, 65.4119) centre (33.5609, 74.9119) ccw
  arc A633 (77.942, 5.6412) -> (75.942, 5.6412) centre (76.942, 5.6412) ccw
  arc A634 (77.9102, 5.6412) -> (77.9737, 5.6412) centre (77.9419, 5.6412) ccw
  arc A635 (75.9102, 5.6412) -> (75.9737, 5.6412) centre (75.9419, 5.6412) ccw
  line L178 (81.4801, 11.4103) -> (81.7411, 11.6191)
  arc A636 (81.753, 11.6042) -> (81.7292, 11.634) centre (81.7411, 11.6191) ccw
  arc A637 (81.4682, 11.4251) -> (81.492, 11.3954) centre (81.4801, 11.4103) ccw
  line L179 (81.7411, 11.6191) -> (81.7411, 10.6793)
  arc A638 (81.7221, 10.6793) -> (81.7602, 10.6793) centre (81.7412, 10.6793) ccw
  arc A639 (81.7602, 11.6191) -> (81.7221, 11.6191) centre (81.7412, 11.6191) ccw
  line L180 (81.4801, 10.6793) -> (82.0022, 10.6793)
  arc A640 (82.0022, 10.6603) -> (82.0022, 10.6984) centre (82.0022, 10.6794) ccw
  arc A641 (81.4801, 10.6984) -> (81.4801, 10.6603) centre (81.4801, 10.6794) ccw
  arc A642 (82.0022, 13.3841) -> (81.7673, 13.6191) centre (81.7672, 13.3841) ccw
  arc A643 (81.9832, 13.3841) -> (82.0213, 13.3841) centre (82.0023, 13.3841) ccw
  arc A644 (81.7673, 13.6382) -> (81.7673, 13.6001) centre (81.7673, 13.6191) ccw
  arc A645 (81.7673, 13.6191) -> (81.4801, 13.4103) centre (81.7672, 13.3173) ccw
  arc A646 (81.7673, 13.6001) -> (81.7673, 13.6381) centre (81.7673, 13.6191) ccw
  arc A647 (81.462, 13.4161) -> (81.4982, 13.4044) centre (81.4801, 13.4103) ccw
  arc A648 (81.9239, 13.2014) -> (82.0022, 13.3841) centre (81.7498, 13.3841) ccw
  arc A649 (81.9107, 13.2152) -> (81.937, 13.1876) centre (81.9239, 13.2014) ccw
  arc A650 (82.0213, 13.3841) -> (81.9832, 13.3842) centre (82.0023, 13.3842) ccw
  line L181 (81.9239, 13.2014) -> (81.4801, 12.6793)
  arc A651 (81.4656, 12.6916) -> (81.4946, 12.667) centre (81.4801, 12.6793) ccw
  arc A652 (81.9384, 13.1891) -> (81.9094, 13.2137) centre (81.9239, 13.2014) ccw
  line L182 (81.4801, 12.6793) -> (82.0022, 12.6793)
  arc A653 (82.0022, 12.6603) -> (82.0022, 12.6984) centre (82.0022, 12.6793) ccw
  arc A654 (81.4801, 12.6984) -> (81.4801, 12.6603) centre (81.4801, 12.6793) ccw
  line L183 (71.9801, 12.6793) -> (72.2411, 12.6793)
  arc A655 (72.2411, 12.6603) -> (72.2411, 12.6984) centre (72.2411, 12.6793) ccw
  arc A656 (71.9801, 12.6984) -> (71.9801, 12.6603) centre (71.9801, 12.6793) ccw
  arc A657 (72.2411, 12.6793) -> (72.2411, 13.2014) centre (72.2411, 12.9404) ccw
  arc A658 (72.2411, 12.6984) -> (72.2411, 12.6603) centre (72.2411, 12.6793) ccw
  arc A659 (72.2411, 13.2205) -> (72.2411, 13.1824) centre (72.2411, 13.2015) ccw
  line L184 (71.9801, 13.6191) -> (72.2934, 13.6191)
  arc A660 (72.2934, 13.6001) -> (72.2934, 13.6382) centre (72.2934, 13.6191) ccw
  arc A661 (71.9801, 13.6382) -> (71.9801, 13.6001) centre (71.9801, 13.6191) ccw
  arc A662 (72.2934, 13.2014) -> (72.2934, 13.6191) centre (72.2934, 13.4103) ccw
  arc A663 (72.2934, 13.2205) -> (72.2934, 13.1824) centre (72.2934, 13.2015) ccw
  arc A664 (72.2934, 13.6382) -> (72.2934, 13.6001) centre (72.2934, 13.6191) ccw
  line L185 (72.2934, 13.2014) -> (72.0845, 13.2014)
  arc A665 (72.0845, 13.2205) -> (72.0845, 13.1824) centre (72.0845, 13.2015) ccw
  arc A666 (72.2934, 13.1824) -> (72.2934, 13.2205) centre (72.2934, 13.2015) ccw
  line L186 (72.1889, 11.6191) -> (71.9801, 10.8881)
  arc A667 (71.9618, 10.8934) -> (71.9984, 10.8829) centre (71.9801, 10.8882) ccw
  arc A668 (72.2073, 11.6139) -> (72.1706, 11.6243) centre (72.189, 11.6191) ccw
  line L187 (71.9801, 10.8881) -> (72.5022, 10.8881)
  arc A669 (72.5022, 10.8691) -> (72.5022, 10.9072) centre (72.5022, 10.8882) ccw
  arc A670 (71.9801, 10.9072) -> (71.9801, 10.8691) centre (71.9801, 10.8882) ccw
  line L188 (72.3456, 11.097) -> (72.3456, 10.6793)
  arc A671 (72.3265, 10.6793) -> (72.3646, 10.6793) centre (72.3456, 10.6793) ccw
  arc A672 (72.3646, 11.097) -> (72.3265, 11.097) centre (72.3456, 11.097) ccw
  arc A673 (76.942, 4.1412) -> (76.942, 20.1412) centre (76.942, 12.1412) ccw
  arc A674 (76.942, 20.1412) -> (76.942, 4.1412) centre (76.942, 12.1412) ccw
  arc A675 (76.942, 5.622) -> (76.942, 18.6604) centre (76.942, 12.1412) ccw
  arc A676 (76.942, 18.6604) -> (76.942, 5.622) centre (76.942, 12.1412) ccw
  arc A677 (76.942, 2.6412) -> (76.942, 21.6412) centre (76.942, 12.1412) ccw
  arc A678 (76.942, 21.6412) -> (76.942, 2.6412) centre (76.942, 12.1412) ccw
  arc A679 (76.8576, 84.3321) -> (76.8576, 65.3321) centre (76.8576, 74.8321) ccw
  line L189 (66.2064, 30.852) -> (46.2064, 30.852)
  arc A680 (46.2064, 30.9028) -> (46.2064, 30.8012) centre (46.2064, 30.852) ccw
  arc A681 (66.2064, 30.8012) -> (66.2064, 30.9028) centre (66.2064, 30.852) ccw
  line L190 (46.2064, 30.852) -> (46.2064, 39.252)
  arc A682 (46.2572, 39.252) -> (46.1556, 39.252) centre (46.2064, 39.252) ccw
  arc A683 (46.1556, 30.852) -> (46.2572, 30.852) centre (46.2064, 30.852) ccw
  line L191 (46.2064, 39.252) -> (50.2684, 39.252)
  arc A684 (50.2684, 39.2012) -> (50.2684, 39.3028) centre (50.2684, 39.252) ccw
  arc A685 (46.2064, 39.3028) -> (46.2064, 39.2012) centre (46.2064, 39.252) ccw
  line L192 (50.2684, 39.252) -> (50.2684, 38.952)
  arc A686 (50.2176, 38.952) -> (50.3192, 38.952) centre (50.2684, 38.952) ccw
  arc A687 (50.3192, 39.252) -> (50.2176, 39.252) centre (50.2684, 39.252) ccw
  line L193 (50.2684, 38.952) -> (51.7474, 38.952)
  arc A688 (51.7474, 38.9012) -> (51.7474, 39.0028) centre (51.7474, 38.952) ccw
  arc A689 (50.2684, 39.0028) -> (50.2684, 38.9012) centre (50.2684, 38.952) ccw
  line L194 (51.7474, 38.952) -> (51.7474, 39.252)
  arc A690 (51.7982, 39.252) -> (51.6966, 39.252) centre (51.7474, 39.252) ccw
  arc A691 (51.6966, 38.952) -> (51.7982, 38.952) centre (51.7474, 38.952) ccw
  line L195 (51.7474, 39.252) -> (54.3234, 39.252)
  arc A692 (54.3234, 39.2012) -> (54.3234, 39.3028) centre (54.3234, 39.252) ccw
  arc A693 (51.7474, 39.3028) -> (51.7474, 39.2012) centre (51.7474, 39.252) ccw
  line L196 (54.3234, 39.252) -> (54.3234, 37.702)
  arc A694 (54.2726, 37.702) -> (54.3742, 37.702) centre (54.3234, 37.702) ccw
  arc A695 (54.3742, 39.252) -> (54.2726, 39.252) centre (54.3234, 39.252) ccw
  line L197 (54.3234, 37.702) -> (58.0894, 37.702)
  arc A696 (58.0894, 37.6512) -> (58.0894, 37.7528) centre (58.0894, 37.702) ccw
  arc A697 (54.3234, 37.7528) -> (54.3234, 37.6512) centre (54.3234, 37.702) ccw
  line L198 (58.0894, 37.702) -> (58.0894, 39.252)
  arc A698 (58.1402, 39.252) -> (58.0386, 39.252) centre (58.0894, 39.252) ccw
  arc A699 (58.0386, 37.702) -> (58.1402, 37.702) centre (58.0894, 37.702) ccw
  line L199 (54.3234, 39.252) -> (58.0894, 39.252)
  arc A700 (58.0894, 39.2012) -> (58.0894, 39.3028) centre (58.0894, 39.252) ccw
  arc A701 (54.3234, 39.3028) -> (54.3234, 39.2012) centre (54.3234, 39.252) ccw
  line L200 (58.0894, 39.252) -> (66.2064, 39.252)
  arc A702 (66.2064, 39.2012) -> (66.2064, 39.3028) centre (66.2064, 39.252) ccw
  arc A703 (58.0894, 39.3028) -> (58.0894, 39.2012) centre (58.0894, 39.252) ccw
  line L201 (66.2064, 39.252) -> (66.2064, 30.852)
  arc A704 (66.1556, 30.852) -> (66.2572, 30.852) centre (66.2064, 30.852) ccw
  arc A705 (66.2572, 39.252) -> (66.1556, 39.252) centre (66.2064, 39.252) ccw
  line L202 (65.0814, 31.777) -> (47.3314, 31.777)
  arc A706 (47.3314, 31.8278) -> (47.3314, 31.7262) centre (47.3314, 31.777) ccw
  arc A707 (65.0814, 31.7262) -> (65.0814, 31.8278) centre (65.0814, 31.777) ccw
  line L203 (47.3314, 31.777) -> (47.3314, 38.327)
  arc A708 (47.3822, 38.327) -> (47.2806, 38.327) centre (47.3314, 38.327) ccw
  arc A709 (47.2806, 31.777) -> (47.3822, 31.777) centre (47.3314, 31.777) ccw
  line L204 (47.3314, 38.327) -> (54.3234, 38.327)
  arc A710 (54.3234, 38.2762) -> (54.3234, 38.3778) centre (54.3234, 38.327) ccw
  arc A711 (47.3314, 38.3778) -> (47.3314, 38.2762) centre (47.3314, 38.327) ccw
  line L205 (58.0894, 38.327) -> (65.0814, 38.327)
  arc A712 (65.0814, 38.2762) -> (65.0814, 38.3778) centre (65.0814, 38.327) ccw
  arc A713 (58.0894, 38.3778) -> (58.0894, 38.2762) centre (58.0894, 38.327) ccw
  line L206 (65.0814, 38.327) -> (65.0814, 31.777)
  arc A714 (65.0306, 31.777) -> (65.1322, 31.777) centre (65.0814, 31.777) ccw
  arc A715 (65.1322, 38.327) -> (65.0306, 38.327) centre (65.0814, 38.327) ccw
  arc A716 (11.0927, 81.3321) -> (13.0927, 81.3321) centre (12.0927, 81.3321) ccw
  arc A717 (11.1245, 81.3321) -> (11.061, 81.3321) centre (11.0928, 81.3321) ccw
  arc A718 (13.1245, 81.3321) -> (13.061, 81.3321) centre (13.0927, 81.3321) ccw
  line L207 (6.5325, 75.5852) -> (6.7936, 75.794)
  arc A719 (6.8055, 75.7791) -> (6.7817, 75.8089) centre (6.7936, 75.794) ccw
  arc A720 (6.5206, 75.6) -> (6.5444, 75.5703) centre (6.5325, 75.5851) ccw
  line L208 (6.7936, 75.794) -> (6.7936, 74.8542)
  arc A721 (6.7745, 74.8542) -> (6.8126, 74.8542) centre (6.7936, 74.8542) ccw
  arc A722 (6.8126, 75.794) -> (6.7745, 75.794) centre (6.7936, 75.794) ccw
  line L209 (6.5325, 74.8542) -> (7.0546, 74.8542)
  arc A723 (7.0546, 74.8352) -> (7.0546, 74.8732) centre (7.0546, 74.8542) ccw
  arc A724 (6.5325, 74.8732) -> (6.5325, 74.8352) centre (6.5325, 74.8542) ccw
  arc A725 (10.0546, 70.559) -> (9.8197, 70.794) centre (9.8196, 70.559) ccw
  arc A726 (10.0356, 70.559) -> (10.0737, 70.559) centre (10.0547, 70.559) ccw
  arc A727 (9.8197, 70.813) -> (9.8197, 70.775) centre (9.8197, 70.794) ccw
  arc A728 (9.8197, 70.794) -> (9.5325, 70.5852) centre (9.8196, 70.4922) ccw
  arc A729 (9.8197, 70.775) -> (9.8197, 70.813) centre (9.8197, 70.794) ccw
  arc A730 (9.5144, 70.591) -> (9.5506, 70.5793) centre (9.5325, 70.5851) ccw
  arc A731 (9.9763, 70.3763) -> (10.0546, 70.559) centre (9.8022, 70.559) ccw
  arc A732 (9.9632, 70.3901) -> (9.9895, 70.3625) centre (9.9764, 70.3763) ccw
  arc A733 (10.0737, 70.559) -> (10.0356, 70.5591) centre (10.0547, 70.559) ccw
  line L210 (9.9763, 70.3763) -> (9.5325, 69.8542)
  arc A734 (9.518, 69.8665) -> (9.547, 69.8419) centre (9.5325, 69.8542) ccw
  arc A735 (9.9908, 70.364) -> (9.9618, 70.3886) centre (9.9763, 70.3763) ccw
  line L211 (9.5325, 69.8542) -> (10.0546, 69.8542)
  arc A736 (10.0546, 69.8352) -> (10.0546, 69.8732) centre (10.0546, 69.8542) ccw
  arc A737 (9.5325, 69.8732) -> (9.5325, 69.8352) centre (9.5325, 69.8542) ccw
  line L212 (12.5325, 74.8542) -> (12.7936, 74.8542)
  arc A738 (12.7936, 74.8352) -> (12.7936, 74.8732) centre (12.7936, 74.8542) ccw
  arc A739 (12.5325, 74.8732) -> (12.5325, 74.8352) centre (12.5325, 74.8542) ccw
  arc A740 (12.7936, 74.8542) -> (12.7936, 75.3763) centre (12.7936, 75.1153) ccw
  arc A741 (12.7936, 74.8732) -> (12.7936, 74.8352) centre (12.7936, 74.8542) ccw
  arc A742 (12.7936, 75.3954) -> (12.7936, 75.3573) centre (12.7936, 75.3764) ccw
  line L213 (12.5325, 75.794) -> (12.8458, 75.794)
  arc A743 (12.8458, 75.775) -> (12.8458, 75.813) centre (12.8458, 75.794) ccw
  arc A744 (12.5325, 75.813) -> (12.5325, 75.775) centre (12.5325, 75.794) ccw
  arc A745 (12.8458, 75.3763) -> (12.8458, 75.794) centre (12.8458, 75.5851) ccw
  arc A746 (12.8458, 75.3954) -> (12.8458, 75.3573) centre (12.8458, 75.3764) ccw
  arc A747 (12.8458, 75.813) -> (12.8458, 75.775) centre (12.8458, 75.794) ccw
  line L214 (12.8458, 75.3763) -> (12.637, 75.3763)
  arc A748 (12.637, 75.3954) -> (12.637, 75.3573) centre (12.637, 75.3764) ccw
  arc A749 (12.8458, 75.3573) -> (12.8458, 75.3954) centre (12.8458, 75.3764) ccw
  arc A750 (12.0927, 66.8321) -> (12.0927, 82.8321) centre (12.0927, 74.8321) ccw
  arc A751 (12.0927, 82.8321) -> (12.0927, 66.8321) centre (12.0927, 74.8321) ccw
  arc A752 (12.0927, 68.3129) -> (12.0927, 81.3513) centre (12.0927, 74.8321) ccw
  arc A753 (12.0927, 81.3513) -> (12.0927, 68.3129) centre (12.0927, 74.8321) ccw
  arc A754 (12.0927, 65.3321) -> (12.0927, 84.3321) centre (12.0927, 74.8321) ccw
  arc A755 (12.0927, 84.3321) -> (12.0927, 65.3321) centre (12.0927, 74.8321) ccw
  arc A756 (99.4424, 47.4569) -> (97.4424, 47.4569) centre (98.4424, 47.4569) ccw
  arc A757 (99.4106, 47.4569) -> (99.4741, 47.4569) centre (99.4424, 47.4569) ccw
  arc A758 (97.4106, 47.4569) -> (97.4741, 47.4569) centre (97.4424, 47.4569) ccw
  line L215 (101.4805, 50.726) -> (101.7415, 50.9348)
  arc A759 (101.7534, 50.9199) -> (101.7296, 50.9497) centre (101.7415, 50.9348) ccw
  arc A760 (101.4686, 50.7408) -> (101.4924, 50.7111) centre (101.4805, 50.7259) ccw
  line L216 (101.7415, 50.9348) -> (101.7415, 49.995)
  arc A761 (101.7225, 49.995) -> (101.7606, 49.995) centre (101.7415, 49.995) ccw
  arc A762 (101.7606, 50.9348) -> (101.7225, 50.9348) centre (101.7415, 50.9348) ccw
  line L217 (101.4805, 49.995) -> (102.0026, 49.995)
  arc A763 (102.0026, 49.976) -> (102.0026, 50.0141) centre (102.0026, 49.995) ccw
  arc A764 (101.4805, 50.0141) -> (101.4805, 49.976) centre (101.4805, 49.995) ccw
  arc A765 (96.0026, 50.6999) -> (95.7676, 50.9348) centre (95.7676, 50.6998) ccw
  arc A766 (95.9835, 50.6999) -> (96.0216, 50.6999) centre (96.0026, 50.6999) ccw
  arc A767 (95.7676, 50.9539) -> (95.7676, 50.9158) centre (95.7676, 50.9349) ccw
  arc A768 (95.7676, 50.9348) -> (95.4805, 50.726) centre (95.7676, 50.633) ccw
  arc A769 (95.7676, 50.9158) -> (95.7676, 50.9539) centre (95.7676, 50.9349) ccw
  arc A770 (95.4623, 50.7318) -> (95.4986, 50.7201) centre (95.4805, 50.7259) ccw
  arc A771 (95.9243, 50.5171) -> (96.0026, 50.6999) centre (95.7501, 50.6999) ccw
  arc A772 (95.9111, 50.5309) -> (95.9374, 50.5033) centre (95.9243, 50.5171) ccw
  arc A773 (96.0216, 50.6999) -> (95.9835, 50.6999) centre (96.0026, 50.6999) ccw
  line L218 (95.9243, 50.5171) -> (95.4805, 49.995)
  arc A774 (95.466, 50.0074) -> (95.495, 49.9827) centre (95.4805, 49.995) ccw
  arc A775 (95.9388, 50.5048) -> (95.9098, 50.5295) centre (95.9243, 50.5172) ccw
  line L219 (95.4805, 49.995) -> (96.0026, 49.995)
  arc A776 (96.0026, 49.976) -> (96.0026, 50.0141) centre (96.0026, 49.995) ccw
  arc A777 (95.4805, 50.0141) -> (95.4805, 49.976) centre (95.4805, 49.995) ccw
  arc A778 (98.4424, 45.9569) -> (98.4424, 61.9569) centre (98.4424, 53.9569) ccw
  arc A779 (98.4424, 61.9569) -> (98.4424, 45.9569) centre (98.4424, 53.9569) ccw
  arc A780 (98.4424, 47.4377) -> (98.4424, 60.4761) centre (98.4424, 53.9569) ccw
  arc A781 (98.4424, 60.4761) -> (98.4424, 47.4377) centre (98.4424, 53.9569) ccw
  arc A782 (98.4424, 44.4569) -> (98.4424, 63.4569) centre (98.4424, 53.9569) ccw
  arc A783 (98.4424, 63.4569) -> (98.4424, 44.4569) centre (98.4424, 53.9569) ccw
  line L220 (82.5754, 38.7985) -> (82.5754, 37.4015)
  arc A784 (82.5373, 37.4015) -> (82.6135, 37.4015) centre (82.5754, 37.4015) ccw
  arc A785 (82.6135, 38.7985) -> (82.5373, 38.7985) centre (82.5754, 38.7985) ccw
  line L221 (72.4154, 31.3055) -> (82.5754, 31.3055)
  arc A786 (82.5754, 31.2674) -> (82.5754, 31.3436) centre (82.5754, 31.3055) ccw
  arc A787 (72.4154, 31.3436) -> (72.4154, 31.2674) centre (72.4154, 31.3055) ccw
  line L222 (72.4154, 31.3055) -> (72.4154, 33.0835)
  arc A788 (72.4535, 33.0835) -> (72.3773, 33.0835) centre (72.4154, 33.0835) ccw
  arc A789 (72.3773, 31.3055) -> (72.4535, 31.3055) centre (72.4154, 31.3055) ccw
  line L223 (82.5754, 38.7985) -> (72.4154, 38.7985)
  arc A790 (72.4154, 38.8366) -> (72.4154, 38.7604) centre (72.4154, 38.7985) ccw
  arc A791 (82.5754, 38.7604) -> (82.5754, 38.8366) centre (82.5754, 38.7985) ccw
  line L224 (82.5754, 32.1945) -> (83.0834, 32.0675)
  arc A792 (83.0742, 32.0305) -> (83.0926, 32.1045) centre (83.0834, 32.0675) ccw
  arc A793 (82.5846, 32.2315) -> (82.5662, 32.1575) centre (82.5754, 32.1945) ccw
  line L225 (82.5754, 32.1945) -> (82.5754, 31.3055)
  arc A794 (82.5373, 31.3055) -> (82.6135, 31.3055) centre (82.5754, 31.3055) ccw
  arc A795 (82.6135, 32.1945) -> (82.5373, 32.1945) centre (82.5754, 32.1945) ccw
  line L226 (83.0834, 32.0675) -> (83.0834, 33.2105)
  arc A796 (83.1215, 33.2105) -> (83.0453, 33.2105) centre (83.0834, 33.2105) ccw
  arc A797 (83.0453, 32.0675) -> (83.1215, 32.0675) centre (83.0834, 32.0675) ccw
  line L227 (83.0834, 33.2105) -> (82.5754, 33.0835)
  arc A798 (82.5662, 33.1205) -> (82.5846, 33.0465) centre (82.5754, 33.0835) ccw
  arc A799 (83.0926, 33.1735) -> (83.0742, 33.2475) centre (83.0834, 33.2105) ccw
  line L228 (82.5754, 33.0835) -> (82.5754, 32.1945)
  arc A800 (82.5373, 32.1945) -> (82.6135, 32.1945) centre (82.5754, 32.1945) ccw
  arc A801 (82.6135, 33.0835) -> (82.5373, 33.0835) centre (82.5754, 33.0835) ccw
  line L229 (82.5754, 33.0835) -> (72.4154, 33.0835)
  arc A802 (72.4154, 33.1216) -> (72.4154, 33.0454) centre (72.4154, 33.0835) ccw
  arc A803 (82.5754, 33.0454) -> (82.5754, 33.1216) centre (82.5754, 33.0835) ccw
  line L230 (72.4154, 33.0835) -> (72.4154, 37.4015)
  arc A804 (72.4535, 37.4015) -> (72.3773, 37.4015) centre (72.4154, 37.4015) ccw
  arc A805 (72.3773, 33.0835) -> (72.4535, 33.0835) centre (72.4154, 33.0835) ccw
  line L231 (82.5754, 37.4015) -> (72.4154, 37.4015)
  arc A806 (72.4154, 37.4396) -> (72.4154, 37.3634) centre (72.4154, 37.4015) ccw
  arc A807 (82.5754, 37.3634) -> (82.5754, 37.4396) centre (82.5754, 37.4015) ccw
  line L232 (82.5754, 37.4015) -> (82.5754, 33.0835)
  arc A808 (82.5373, 33.0835) -> (82.6135, 33.0835) centre (82.5754, 33.0835) ccw
  arc A809 (82.6135, 37.4015) -> (82.5373, 37.4015) centre (82.5754, 37.4015) ccw
  line L233 (72.4154, 37.4015) -> (72.4154, 38.7985)
  arc A810 (72.4535, 38.7985) -> (72.3773, 38.7985) centre (72.4154, 38.7985) ccw
  arc A811 (72.3773, 37.4015) -> (72.4535, 37.4015) centre (72.4154, 37.4015) ccw
  line L234 (81.3971, 32.4471) -> (81.637, 32.639)
  arc A812 (81.6568, 32.6142) -> (81.6172, 32.6638) centre (81.637, 32.639) ccw
  arc A813 (81.3773, 32.4719) -> (81.417, 32.4223) centre (81.3972, 32.4471) ccw
  line L235 (81.637, 32.639) -> (81.637, 31.7754)
  arc A814 (81.6053, 31.7754) -> (81.6688, 31.7754) centre (81.6371, 31.7754) ccw
  arc A815 (81.6688, 32.639) -> (81.6053, 32.639) centre (81.6371, 32.639) ccw
  line L236 (81.3971, 31.7754) -> (81.8769, 31.7754)
  arc A816 (81.8769, 31.7437) -> (81.8769, 31.8072) centre (81.8769, 31.7755) ccw
  arc A817 (81.3971, 31.8072) -> (81.3971, 31.7437) centre (81.3971, 31.7755) ccw
  arc A818 (76.7969, 32.4231) -> (76.581, 32.639) centre (76.581, 32.4231) ccw
  arc A819 (76.7652, 32.4231) -> (76.8287, 32.4231) centre (76.7969, 32.4231) ccw
  arc A820 (76.581, 32.6708) -> (76.581, 32.6073) centre (76.581, 32.639) ccw
  arc A821 (76.581, 32.639) -> (76.3171, 32.4471) centre (76.581, 32.3616) ccw
  arc A822 (76.581, 32.6073) -> (76.581, 32.6707) centre (76.581, 32.639) ccw
  arc A823 (76.2869, 32.4569) -> (76.3473, 32.4373) centre (76.3171, 32.4471) ccw
  arc A824 (76.7249, 32.2552) -> (76.7969, 32.4231) centre (76.5651, 32.4231) ccw
  arc A825 (76.703, 32.2782) -> (76.7468, 32.2322) centre (76.7249, 32.2552) ccw
  arc A826 (76.8286, 32.4231) -> (76.7652, 32.4231) centre (76.7969, 32.4231) ccw
  line L237 (76.7249, 32.2552) -> (76.3171, 31.7754)
  arc A827 (76.2929, 31.796) -> (76.3413, 31.7548) centre (76.3171, 31.7754) ccw
  arc A828 (76.7491, 32.2346) -> (76.7007, 32.2757) centre (76.7249, 32.2552) ccw
  line L238 (76.3171, 31.7754) -> (76.7969, 31.7754)
  arc A829 (76.7969, 31.7437) -> (76.7969, 31.8072) centre (76.7969, 31.7755) ccw
  arc A830 (76.3171, 31.8072) -> (76.3171, 31.7437) centre (76.3171, 31.7754) ccw
  arc A831 (74.9808, 31.6865) -> (74.9808, 32.7025) centre (74.9808, 32.1945) ccw
  arc A832 (74.9808, 32.7025) -> (74.9808, 31.6865) centre (74.9808, 32.1945) ccw